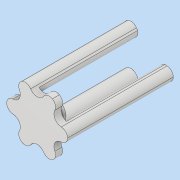
# Autodesk Inventor part: FixedCylinderWireStorageInsert
Saved by Autodesk Inventor 2017 (Build 210142000, 142)
## iProperties
Created: 2016-12-15
Part Number: FixedCylinderWireStorageInsert
Material: ABS Plastic
Document SubType Name: Modeling
Designer: techn
Density: 1.06 g/cm^3
Appearance: Smooth - White
Author: techn
Autodesk Inventor part; units mm, degrees
ref_plane "YZ Plane" through (0, 0, 0) normal (1, 0, 0) x (0, 1, 0)
ref_plane "XZ Plane" through (0, 0, 0) normal (0, 1, 0) x (-1, 0, 0)
ref_plane "XY Plane" through (0, 0, 0) normal (0, 0, 1) x (1, 0, 0)
sketch "Sketch2" plane through (0, 0, 0) normal (0, 0, 1) x (1, 0, 0)
  arc A0 (8.1994, 7.8486) -> (6.9887, 12.0963) centre (5.4003, 9.3471) ccw
  arc A1 (6.9887, 12.0963) -> (6.9813, 12.1005) centre (0, 0) ccw
  arc A2 (6.9813, 12.1005) -> (2.6973, 11.0252) centre (5.3947, 9.3504) ccw
  arc A3 (-2.6973, 11.0252) -> (2.6973, 11.0252) centre (0, 12.7) ccw
  arc A4 (-2.6973, 11.0252) -> (-6.9813, 12.1005) centre (-5.3947, 9.3504) ccw
  arc A5 (-6.9813, 12.1005) -> (-6.9887, 12.0963) centre (0, 0) ccw
  arc A6 (-6.9887, 12.0963) -> (-8.1994, 7.8486) centre (-5.4003, 9.3471) ccw
  arc A7 (-10.8968, 3.1766) -> (-8.1994, 7.8486) centre (-10.9985, 6.35) ccw
  arc A8 (-10.8968, 3.1766) -> (-13.97, 0.0042) centre (-10.795, 0.0033) ccw
  arc A9 (-13.97, 0.0042) -> (-13.97, -0.0042) centre (0, 0) ccw
  arc A10 (-13.97, -0.0042) -> (-10.8968, -3.1766) centre (-10.795, -0.0033) ccw
  arc A11 (-8.1994, -7.8486) -> (-10.8968, -3.1766) centre (-10.9985, -6.35) ccw
  arc A12 (-8.1994, -7.8486) -> (-6.9887, -12.0963) centre (-5.4003, -9.3471) ccw
  arc A13 (-6.9887, -12.0963) -> (-6.9813, -12.1005) centre (0, 0) ccw
  arc A14 (-6.9813, -12.1005) -> (-2.6973, -11.0252) centre (-5.3947, -9.3504) ccw
  arc A15 (2.6973, -11.0252) -> (-2.6973, -11.0252) centre (0, -12.7) ccw
  arc A16 (2.6973, -11.0252) -> (6.9813, -12.1005) centre (5.3947, -9.3504) ccw
  arc A17 (6.9813, -12.1005) -> (6.9887, -12.0963) centre (0, 0) ccw
  arc A18 (6.9887, -12.0963) -> (8.1994, -7.8486) centre (5.4003, -9.3471) ccw
  arc A19 (10.8968, -3.1766) -> (8.1994, -7.8486) centre (10.9985, -6.35) ccw
  arc A20 (10.8968, -3.1766) -> (13.97, -0.0042) centre (10.795, -0.0033) ccw
  arc A21 (13.97, -0.0042) -> (13.97, 0.0042) centre (0, 0) ccw
  arc A22 (13.97, 0.0042) -> (10.8968, 3.1766) centre (10.795, 0.0033) ccw
  arc A23 (8.1994, 7.8486) -> (10.8968, 3.1766) centre (10.9985, 6.35) ccw
  circle A24 centre (0, 0) radius 1.5875
  constraints: 48 point on circle, 25 centre point
extrude "Extrusion1" add sketch "Sketch2" against normal blind 3.175 contours A23 A22 A21 A20 A19 A18 A17 A16 A15 A14 A13 A12 A11 A10 A9 A8 A7 A6 A5 A4 A3 A2 A1 A0 | A24
sketch "Sketch3" plane through (0, 0, -3.175) normal (0, 0, -1) x (-1, 0, 0)
  circle A0 centre (0, 0) radius 3.3655
  circle A1 centre (0, 0) radius 4.7625
  dimension "d11" = 6.731
  dimension "d12" = 9.525
  constraints: 2 centre point, 2 coincident
  measures "d11" diameter of A0
  measures "d12" diameter of A1
extrude "Extrusion2" add sketch "Sketch3" along normal blind 5.08
sketch "Sketch4" plane through (0, 0, -3.175) normal (0, 0, -1) x (-1, 0, 0)
  arc A0 (-6.9887, 12.0963) -> (-8.1994, 7.8486) centre (-5.4003, 9.3471) ccw projected
  arc A1 (-10.8968, 3.1766) -> (-8.1994, 7.8486) centre (-10.9985, 6.35) ccw projected
  arc A2 (-10.8968, 3.1766) -> (-13.97, 0.0042) centre (-10.795, 0.0033) ccw projected
  arc A3 (-13.97, 0.0042) -> (-13.97, -0.0042) centre (0, 0) ccw projected
  arc A4 (-13.97, -0.0042) -> (-10.8968, -3.1766) centre (-10.795, -0.0033) ccw projected
  arc A5 (-8.1994, -7.8486) -> (-10.8968, -3.1766) centre (-10.9985, -6.35) ccw projected
  arc A6 (-8.1994, -7.8486) -> (-6.9887, -12.0963) centre (-5.4003, -9.3471) ccw projected
  arc A7 (-6.9887, -12.0963) -> (-6.9813, -12.1005) centre (0, 0) ccw projected
  arc A8 (-6.9813, -12.1005) -> (-2.6973, -11.0252) centre (-5.3947, -9.3504) ccw projected
  arc A9 (2.6973, -11.0252) -> (-2.6973, -11.0252) centre (0, -12.7) ccw projected
  arc A10 (2.6973, -11.0252) -> (6.9813, -12.1005) centre (5.3947, -9.3504) ccw projected
  arc A11 (6.9813, -12.1005) -> (6.9887, -12.0963) centre (0, 0) ccw projected
  arc A12 (6.9887, -12.0963) -> (8.1994, -7.8486) centre (5.4003, -9.3471) ccw projected
  arc A13 (10.8968, -3.1766) -> (8.1994, -7.8486) centre (10.9985, -6.35) ccw projected
  arc A14 (10.8968, -3.1766) -> (13.97, -0.0042) centre (10.795, -0.0033) ccw projected
  arc A15 (13.97, -0.0042) -> (13.97, 0.0042) centre (0, 0) ccw projected
  arc A16 (13.97, 0.0042) -> (10.8968, 3.1766) centre (10.795, 0.0033) ccw projected
  arc A17 (8.1994, 7.8486) -> (10.8968, 3.1766) centre (10.9985, 6.35) ccw projected
  arc A18 (8.1994, 7.8486) -> (6.9887, 12.0963) centre (5.4003, 9.3471) ccw projected
  arc A19 (6.9887, 12.0963) -> (6.9813, 12.1005) centre (0, 0) ccw projected
  arc A20 (6.9813, 12.1005) -> (2.6973, 11.0252) centre (5.3947, 9.3504) ccw projected
  arc A21 (-2.6973, 11.0252) -> (2.6973, 11.0252) centre (0, 12.7) ccw projected
  arc A22 (-2.6973, 11.0252) -> (-6.9813, 12.1005) centre (-5.3947, 9.3504) ccw projected
  arc A23 (-6.9813, 12.1005) -> (-6.9887, 12.0963) centre (0, 0) ccw projected
  circle A24 centre (0, 0) radius 4.7625 projected
  circle A25 centre (-10.795, -0.0033) radius 3.175
  circle A26 centre (5.3947, 9.3504) radius 3.175
  circle A27 centre (5.4003, -9.3471) radius 3.175
  constraints: 3 centre point, 3 coincident, 1 concentric
extrude "Extrusion4" add sketch "Sketch4" along normal blind 44.45 contours A25 A4 A3 | A20 A19 A26 | A27 A12 A11
fillet "Fillet1" radius 3.81 1 edges at (4.7625, 0, -3.175)
sketch "Sketch5" plane through (0, 0, 0) normal (0, 0, 1) x (1, 0, 0)
  arc A0 (8.1994, 7.8486) -> (6.9887, 12.0963) centre (5.4003, 9.3471) ccw projected
  arc A1 (6.9887, 12.0963) -> (6.9813, 12.1005) centre (0, 0) ccw projected
  arc A2 (6.9813, 12.1005) -> (2.6973, 11.0252) centre (5.3947, 9.3504) ccw projected
  arc A3 (-2.6973, 11.0252) -> (2.6973, 11.0252) centre (0, 12.7) ccw projected
  arc A4 (-2.6973, 11.0252) -> (-6.9813, 12.1005) centre (-5.3947, 9.3504) ccw projected
  arc A5 (-6.9813, 12.1005) -> (-6.9887, 12.0963) centre (0, 0) ccw projected
  arc A6 (-6.9887, 12.0963) -> (-8.1994, 7.8486) centre (-5.4003, 9.3471) ccw projected
  arc A7 (-10.8968, 3.1766) -> (-8.1994, 7.8486) centre (-10.9985, 6.35) ccw projected
  arc A8 (-10.8968, 3.1766) -> (-13.97, 0.0042) centre (-10.795, 0.0033) ccw projected
  arc A9 (-13.97, 0.0042) -> (-13.97, -0.0042) centre (0, 0) ccw projected
  arc A10 (-13.97, -0.0042) -> (-10.8968, -3.1766) centre (-10.795, -0.0033) ccw projected
  arc A11 (-8.1994, -7.8486) -> (-10.8968, -3.1766) centre (-10.9985, -6.35) ccw projected
  arc A12 (-8.1994, -7.8486) -> (-6.9887, -12.0963) centre (-5.4003, -9.3471) ccw projected
  arc A13 (-6.9887, -12.0963) -> (-6.9813, -12.1005) centre (0, 0) ccw projected
  arc A14 (-6.9813, -12.1005) -> (-2.6973, -11.0252) centre (-5.3947, -9.3504) ccw projected
  arc A15 (2.6973, -11.0252) -> (-2.6973, -11.0252) centre (0, -12.7) ccw projected
  arc A16 (2.6973, -11.0252) -> (6.9813, -12.1005) centre (5.3947, -9.3504) ccw projected
  arc A17 (6.9813, -12.1005) -> (6.9887, -12.0963) centre (0, 0) ccw projected
  arc A18 (6.9887, -12.0963) -> (8.1994, -7.8486) centre (5.4003, -9.3471) ccw projected
  arc A19 (10.8968, -3.1766) -> (8.1994, -7.8486) centre (10.9985, -6.35) ccw projected
  arc A20 (10.8968, -3.1766) -> (13.97, -0.0042) centre (10.795, -0.0033) ccw projected
  arc A21 (13.97, -0.0042) -> (13.97, 0.0042) centre (0, 0) ccw projected
  arc A22 (13.97, 0.0042) -> (10.8968, 3.1766) centre (10.795, 0.0033) ccw projected
  arc A23 (8.1994, 7.8486) -> (10.8968, 3.1766) centre (10.9985, 6.35) ccw projected
  arc A24 (6.8544, 11.8805) -> (2.9131, 10.8912) centre (5.3947, 9.3504) ccw
  arc A25 (6.8616, 11.8763) -> (6.8544, 11.8805) centre (0, 0) ccw
  arc A26 (7.9755, 7.9684) -> (6.8616, 11.8763) centre (5.4003, 9.3471) ccw
  arc A27 (7.9755, 7.9684) -> (10.8886, 2.9228) centre (10.9985, 6.35) ccw
  arc A28 (13.716, 0.0041) -> (10.8886, 2.9228) centre (10.795, 0.0033) ccw
  arc A29 (13.716, -0.0041) -> (13.716, 0.0041) centre (0, 0) ccw
  arc A30 (10.8886, -2.9228) -> (13.716, -0.0041) centre (10.795, -0.0033) ccw
  arc A31 (10.8886, -2.9228) -> (7.9755, -7.9684) centre (10.9985, -6.35) ccw
  arc A32 (6.8616, -11.8763) -> (7.9755, -7.9684) centre (5.4003, -9.3471) ccw
  arc A33 (6.8544, -11.8805) -> (6.8616, -11.8763) centre (0, 0) ccw
  arc A34 (2.9131, -10.8912) -> (6.8544, -11.8805) centre (5.3947, -9.3504) ccw
  arc A35 (2.9131, -10.8912) -> (-2.9131, -10.8912) centre (0, -12.7) ccw
  arc A36 (-6.8544, -11.8805) -> (-2.9131, -10.8912) centre (-5.3947, -9.3504) ccw
  arc A37 (-6.8616, -11.8763) -> (-6.8544, -11.8805) centre (0, 0) ccw
  arc A38 (-7.9755, -7.9684) -> (-6.8616, -11.8763) centre (-5.4003, -9.3471) ccw
  arc A39 (-7.9755, -7.9684) -> (-10.8886, -2.9228) centre (-10.9985, -6.35) ccw
  arc A40 (-13.716, -0.0041) -> (-10.8886, -2.9228) centre (-10.795, -0.0033) ccw
  arc A41 (-13.716, 0.0041) -> (-13.716, -0.0041) centre (0, 0) ccw
  arc A42 (-10.8886, 2.9228) -> (-13.716, 0.0041) centre (-10.795, 0.0033) ccw
  arc A43 (-10.8886, 2.9228) -> (-7.9755, 7.9684) centre (-10.9985, 6.35) ccw
  arc A44 (-6.8616, 11.8763) -> (-7.9755, 7.9684) centre (-5.4003, 9.3471) ccw
  arc A45 (-6.8544, 11.8805) -> (-6.8616, 11.8763) centre (0, 0) ccw
  arc A46 (-2.9131, 10.8912) -> (-6.8544, 11.8805) centre (-5.3947, 9.3504) ccw
  arc A47 (-2.9131, 10.8912) -> (2.9131, 10.8912) centre (0, 12.7) ccw
  dimension "d20" = 0.254
  constraints: 48 point on circle, 24 centre point, 23 other
  measures "d20" radial gap between concentric circles of A3 A47
extrude "Extrusion5" cut sketch "Sketch5" against normal through all
body "Solid1"
